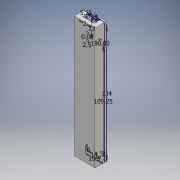
# Autodesk Inventor part: case-bottom
Saved by Autodesk Inventor 2017 (Build 210142000, 142)
## iProperties
Created: 2026-06-28
Part Number: case-bottom
Material: Generic
Document SubType Name: Modeling
Designer: hashire umamusume
Density: 1 g/cm^3
Appearance: Default
Author: hashire umamusume
Autodesk Inventor part; units mm, degrees
ref_plane "YZ Plane" through (0, 0, 0) normal (1, 0, 0) x (0, 1, 0)
ref_plane "XZ Plane" through (0, 0, 0) normal (0, 1, 0) x (-1, 0, 0)
ref_plane "XY Plane" through (0, 0, 0) normal (0, 0, 1) x (1, 0, 0)
sketch "Sketch1" plane through (0, 0, 0) normal (0, 1, 0) x (-1, 0, 0)
  line L0 (0, 0) -> (-19.5, 0)
  line L1 (-19.5, 0) -> (-19.5, -134)
  line L2 (-19.5, -134) -> (0, -134)
  line L3 (0, -134) -> (0, 0)
  line L4 (2, 2) -> (-21.5, 2)
  line L5 (-21.5, 2) -> (-21.5, -136)
  line L6 (-21.5, -136) -> (2, -136)
  line L7 (2, -136) -> (2, 2)
  line L8 (-2.5, -22) -> (-16.5, -22)
  line L9 (-16.5, -22) -> (-16.5, -131.25)
  line L10 (-16.5, -131.25) -> (-2.5, -131.25)
  line L11 (-2.5, -131.25) -> (-2.5, -22)
  line L12 (-2.5, -22) -> (0, -22)
  line L13 (-2.5, -22) -> (0, -22) construction
  line L14 (-16.5, -22) -> (-19.5, -22)
  line L15 (-16.5, -22) -> (-13.5, -22) construction
  line L16 (-6.724, -131.25) -> (-3.974, -131.25) construction
  line L17 (-6, -131.25) -> (-6, -134)
  line L18 (-2.5, -128) -> (0, -128)
  line L19 (-3.25, 2) -> (-16.25, 2)
  line L20 (-16.25, 2) -> (-16.25, 0)
  line L21 (-16.25, 0) -> (-3.25, 0)
  line L22 (-3.25, 0) -> (-3.25, 2)
  line L23 (-19.5, 0) -> (-21.5, 0)
  line L24 (-21.5, 0) -> (-21.5, 2)
  line L25 (-21.5, 2) -> (-19.5, 2)
  line L26 (-19.5, 2) -> (-19.5, 0)
  line L27 (0, 0) -> (2, 0)
  line L28 (2, 0) -> (2, 2)
  line L29 (2, 2) -> (0, 2)
  line L30 (0, 2) -> (0, 0)
  line L31 (0, -134) -> (2, -134)
  line L32 (2, -134) -> (2, -136)
  line L33 (2, -136) -> (0, -136)
  line L34 (0, -136) -> (0, -134)
  line L35 (-19.5, -134) -> (-21.5, -134)
  line L36 (-21.5, -134) -> (-21.5, -136)
  line L37 (-21.5, -136) -> (-19.5, -136)
  line L38 (-19.5, -136) -> (-19.5, -134)
  dimension "d0" = 19.5
  dimension "d1" = 134
  dimension "d2" = 2
  dimension "d3" = 2
  dimension "d4" = 2
  dimension "d5" = 2
  dimension "d6" = 14
  dimension "d7" = 109.25
  dimension "d8" = 22
  dimension "d9" = 2.5
  dimension "d10" = 0
  dimension "d11" = 180
  dimension "d17" = 6
  dimension "d18" = 6
  dimension "d20" = 13
  dimension "d21" = 5.25
  constraints: 78 end point, 16 parallel, 11 horizontal, 10 perpendicular, 9 point on line, 2 collinear
  measures "d0" distance of L2.end L1.end
  measures "d1" distance of L1.end L0.end
  measures "d2" distance between parallel lines of L6 L2
  measures "d3" distance between parallel lines of L1 L5
  measures "d4" distance between parallel lines of L0 L4
  measures "d5" distance between parallel lines of L3 L7
  measures "d6" distance of L10.end L9.end
  measures "d7" distance of L9.end L8.end
  measures "d8" distance between parallel lines of L8 L0
  measures "d9" distance between parallel lines of L3 L11
  measures "d10" distance between parallel lines of L12 L13
  measures "d11" angle of L14 L15
  measures "d17" distance between parallel lines of L3 L17
  measures "d18" distance between parallel lines of L2 L18
  measures "d20" distance between parallel lines of L22 L20
  measures "d21" distance between parallel lines of L7 L22
extrude "Extrusion1" add sketch "Sketch1" against normal blind 11
extrude "Extrusion2" cut sketch "Sketch1" against normal blind 10 contours L3 L12 L8 L14 L1 L0 | L3 L2 L17 L10 L11 L18 | L11 L10 L9 L8
fillet "Fillet1" radius 1 4 edges at (2.5, -5, -128) (1.25, 0, -128) (6, 0, -132.625) (6, -5, -131.25)
extrude "Extrusion3" cut sketch "Sketch1" against normal blind 7 contours L0 L20 L4 L22
extrude "Extrusion4" add sketch "Sketch1" along normal blind 2 contours L27 L7 L31 L3 | L30 L4 L7 L27 | L0 L22 L4 L30 | L0 L26 L4 L20 | L7 L6 L34 L31 | L1 L35 L5 L23 | L23 L5 L4 L26 | L34 L6 L38 L2 | L38 L6 L5 L35
body "Solid1"
